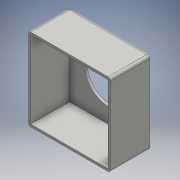
# Autodesk Inventor part: Top
Saved by Autodesk Inventor 2016 (Build 200138000, 138)
## iProperties
Created: 2015-11-09
Part Number: Top
Material: Generic
Document SubType Name: Modeling
Designer: Sudhar
Density: 1 g/cm^3
Appearance: Default
Author: Sudhar
Autodesk Inventor part; units mm, degrees
ref_plane "YZ Plane" through (0, 0, 0) normal (1, 0, 0) x (0, 1, 0)
ref_plane "XZ Plane" through (0, 0, 0) normal (0, 1, 0) x (-1, 0, 0)
ref_plane "XY Plane" through (0, 0, 0) normal (0, 0, 1) x (1, 0, 0)
sketch "Sketch1" plane through (0, 0, 0) normal (0, 1, 0) x (-1, 0, 0)
  line L0 (50.3036, 45.5466) -> (-49.6964, 45.5466)
  line L1 (-49.6964, 45.5466) -> (-49.6964, -54.4534)
  line L2 (-49.6964, -54.4534) -> (50.3036, -54.4534)
  line L3 (50.3036, -54.4534) -> (50.3036, 45.5466)
  point P0 (0, 0)
  dimension "d0" = 100
  dimension "d1" = 100
  constraints: 8 end point, 2 parallel, 1 horizontal, 1 perpendicular
  measures "d0" distance of L2.end L0.start
  measures "d1" distance of L1.end L2.end
extrude "Extrusion1" add sketch "Sketch1" along normal blind 50
fillet "Fillet1" radius 3 8 edges at (49.6964, 50, -4.4534) (-0.3036, 50, 45.5466) (49.6964, 25, 45.5466) (-50.3036, 25, 45.5466) (-50.3036, 50, -4.4534) (-0.3036, 50, -54.4534) (49.6964, 25, -54.4534) (-50.3036, 25, -54.4534)
shell "Shell1" thickness 3 removed faces 1 at (14.363, 0, 11.2132)
sketch "Sketch2" plane through (0, 50, 0) normal (0, 1, 0) x (1, 0, 0)
  circle A0 centre (-0.3036, 4.4534) radius 28
  line L0 (-47.3036, -45.5466) -> (46.6964, -45.5466) projected
  line L1 (-50.3036, 51.4534) -> (-50.3036, -42.5466) projected
  point P0 (0, 0)
  dimension "d6" = 56
  dimension "d7" = 50
  dimension "d8" = 50
  constraints: 1 centre point
  measures "d6" diameter of A0
  measures "d7" distance from line of A0.centre L0
  measures "d8" distance from line of A0.centre L1
extrude "Extrusion2" cut sketch "Sketch2" against normal blind 50
body "Solid1"
